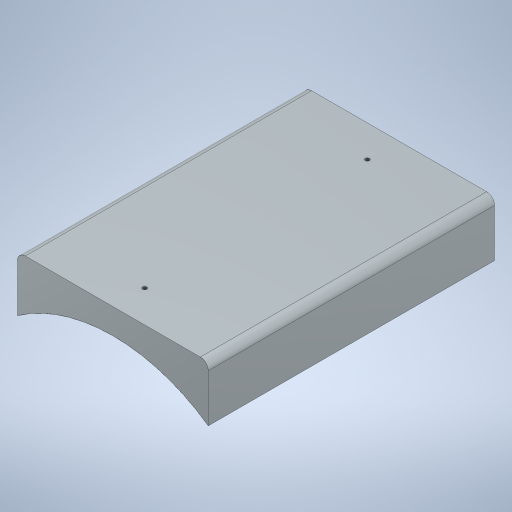
# Autodesk Inventor part: NEW Dudukan di Bearring
Saved by Autodesk Inventor 2023 (Build 270158000, 158)
## iProperties
Created: 2023-10-27
Part Number: NEW Dudukan di Bearring
Material: Generic
Document SubType Name: Modeling
Designer: pms11
Density: 1 g/cm^3
Appearance: Zinc
Author: pms11
Autodesk Inventor part; units mm, degrees
ref_plane "YZ Plane" through (0, 0, 0) normal (1, 0, 0) x (0, 1, 0)
ref_plane "XZ Plane" through (0, 0, 0) normal (0, 1, 0) x (-1, 0, 0)
ref_plane "XY Plane" through (0, 0, 0) normal (0, 0, 1) x (1, 0, 0)
sketch "Sketch1" plane through (0, 0, 0) normal (0, 0, 1) x (1, 0, 0)
  arc A0 (60, 0) -> (-60, 0) centre (0, -84.947) ccw
  line L0 (60, 0) -> (60, 30)
  line L1 (60, 30) -> (60, 35)
  line L2 (-60, 35) -> (-60, 0)
  line L3 (60, 35) -> (-60, 35)
  point P0 (0, 0)
  dimension "d2" = 104
  dimension "d9" = 30
  dimension "d10" = 5
  constraints: 8 end point, 2 point on circle, 1 centre point, 1 vertical
  measures "d2" radius of A0
  measures "d9" distance of L0.start L0.end
  measures "d10" distance of L0.end L1.end
extrude "Extrusion1" add sketch "Sketch1" along normal blind 180
fillet "Fillet5" radius 5 2 edges at (-60, 35, 90) (60, 35, 90)
sketch "Sketch5" plane through (-55, 35, 0) normal (0, 1, 0) x (1, 0, 0)
  line L0 (115, -180) -> (-5, -180) projected
  circle A0 centre (55, -160) radius 1.25
  circle A1 centre (55, -20) radius 1.25
  point P0 (55, 0)
  constraints: 2 centre point
extrude "Extrusion5" cut sketch "Sketch5" against normal blind 3
thread "Thread4" size "M2.5x0.45" class "6H" standard "ANSI Metric M Profile" full length
thread "Thread5" size "M2.5x0.45" class "6H" standard "ANSI Metric M Profile" full length
body "Solid1"
